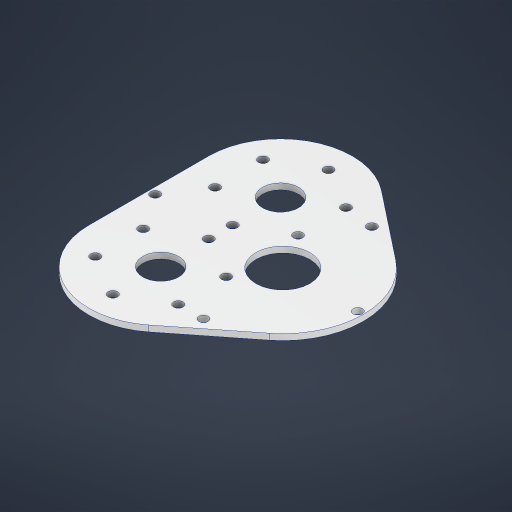
# Autodesk Inventor part: Gearboxes_3_thingy that holds motors and more
Saved by Autodesk Inventor 2024.4 (Build 284460000, 460)
## iProperties
Created: 2026-06-11
Part Number: Gearboxes_3_thingy that holds motors and more
Material: Aluminum 6061
Document SubType Name: Modeling
Designer: stanr
Density: 2.7 g/cm^3
Appearance: Aluminum - Flat
Author: stanr
Autodesk Inventor part; units mm, degrees
ref_plane "YZ Plane" through (0, 0, 0) normal (1, 0, 0) x (0, 1, 0)
ref_plane "XZ Plane" through (0, 0, 0) normal (0, 1, 0) x (-1, 0, 0)
ref_plane "XY Plane" through (0, 0, 0) normal (0, 0, 1) x (1, 0, 0)
sketch "Sketch1" plane through (0, 0, 0) normal (0, 1, 0) x (-1, 0, 0)
  circle A0 centre (0, 0) radius 31.75 construction
  circle A1 centre (0, -63.5) radius 31.75 construction
  circle A2 centre (0, 0) radius 9.525
  circle A3 centre (0, -63.5) radius 9.525
  circle A4 centre (0, 0) radius 25.4 construction
  circle A5 centre (0, -63.5) radius 25.4 construction
  circle A6 centre (0, 25.4) radius 2.4892
  circle A7 centre (-21.997, 12.7) radius 2.4892
  circle A8 centre (-21.997, -12.7) radius 2.4892
  circle A9 centre (0, -25.4) radius 2.4892
  circle A10 centre (21.997, -12.7) radius 2.4892
  circle A11 centre (21.997, 12.7) radius 2.4892
  circle A12 centre (0, -88.9) radius 2.4892
  circle A13 centre (21.997, -76.2) radius 2.4892
  circle A14 centre (21.997, -50.8) radius 2.4892
  circle A15 centre (0, -38.1) radius 2.4892
  circle A16 centre (-21.997, -50.8) radius 2.4892
  circle A17 centre (-21.997, -76.2) radius 2.4892
  circle A18 centre (-32.9859, -31.75) radius 36.2585 construction
  circle A19 centre (-32.9859, -31.75) radius 14.2875
  line L0 (31.75, 0) -> (31.75, -63.5) construction
  line L1 (38.1, -14.6551) -> (38.1, -63.5)
  arc A20 (-23.5901, -93.4185) -> (38.1, -63.5) centre (0, -63.5) ccw
  line L2 (-19.6584, -88.4321) -> (-55.4358, -60.2225) construction
  arc A21 (-55.4358, -3.2775) -> (-55.4358, -60.2225) centre (-32.9859, -31.75) ccw construction
  line L3 (-19.6584, 24.9321) -> (-55.4358, -3.2775) construction
  line L4 (-23.5901, 29.9185) -> (-59.3674, 1.7089)
  line L5 (-23.5901, -93.4185) -> (-59.3674, -65.2089)
  arc A22 (-59.3674, 1.7089) -> (-59.3674, -65.2089) centre (-32.9859, -31.75) ccw
  arc A23 (31.75, 0) -> (-19.6584, 24.9321) centre (0, 0) ccw
  arc A24 (38.1, 0) -> (-23.5901, 29.9185) centre (0, 0) ccw
  line L6 (38.1, 0) -> (38.1, -63.8348)
  circle A25 centre (34.671, -31.75) radius 2.4892
  circle A26 centre (-35.2871, 12.6092) radius 2.4892
  circle A27 centre (-37.5471, -74.3273) radius 2.4892
  circle A28 centre (-72.6734, -31.75) radius 2.4892
  circle A29 centre (-35.2871, 12.6092) radius 3.175 construction
  circle A30 centre (-72.6734, -31.75) radius 3.175 construction
  circle A31 centre (34.671, -31.75) radius 3.175 construction
  point P0 (38.1, -14.6551)
  point P1 (-75.5944, -31.75)
  dimension "d4" = 50.8
  dimension "d0" = 63.5
  dimension "d2" = 19.05
  dimension "d5" = 4.9784
  dimension "d8" = 360
  dimension "d12" = 360
  dimension "d14" = 72.517
  dimension "d15" = 28.575
  dimension "d16" = 6.35
  dimension "d20" = 6.35
  dimension "d23" = 6.35
  dimension "d24" = 66.8482
  dimension "d25" = 105.4672
  dimension "d28" = 4.9784
  dimension "d29" = 2.921
  dimension "d30" = 4.9784
  dimension "d31" = 37.4723
  dimension "d32" = 4.9784
  dimension "d33" = 4.9784
  dimension "d34" = 2.921
  dimension "d35" = 6.35
  dimension "d36" = 6.35
  dimension "d37" = 6.35
  dimension "d38" = 45.7835
  constraints: 30 centre point, 17 point on circle, 14 end point, 13 tangent, 10 coincident, 5 equal radius, 5 vertical alignment, 3 horizontal alignment, 2 parallel, 1 midpoint, 1 point on line, 32 other
  measures "d0" diameter of A0
  measures "d2" diameter of A2
  measures "d5" diameter of A6
  measures "d14" diameter of A18
  measures "d15" diameter of A19
  measures "d16" distance between parallel lines of L0 L1
  measures "d20" distance between parallel lines of L3 L4
  measures "d23" radial gap between concentric circles of A1 A20
  measures "d24" distance from line of L1.start L3
  measures "d25" distance from line of L6.end L3
  measures "d28" diameter of A25
  measures "d29" distance from line of L0 A25.centre
  measures "d30" diameter of A26
  measures "d31" distance of A0.centre A26.centre
  measures "d32" diameter of A27
  measures "d33" diameter of A28
  measures "d34" distance of point (-75.594, -31.75) A28.centre
  measures "d35" diameter of A29
  measures "d36" diameter of A30
  measures "d37" diameter of A31
  measures "d38" distance of point (0, 0) A18.centre
extrude "Extrusion1" add sketch "Sketch1" along normal blind 3.175
equation "\"d29\" = d34"
body "Solid1"
